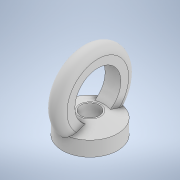
# Autodesk Inventor part: Wire holder
Saved by Autodesk Inventor 2020.2 (Build 242310000, 310)
## iProperties
Created: 2020-01-20
Part Number: Wire holder
Material: Generic
Document SubType Name: Modeling
Designer: Paul Lefeuvre
Density: 1 g/cm^3
Appearance: Default
Author: Paul Lefeuvre
Autodesk Inventor part; units mm, degrees
ref_plane "YZ Plane" through (0, 0, 0) normal (1, 0, 0) x (0, 1, 0)
ref_plane "XZ Plane" through (0, 0, 0) normal (0, 1, 0) x (-1, 0, 0)
ref_plane "XY Plane" through (0, 0, 0) normal (0, 0, 1) x (1, 0, 0)
sketch "Sketch1" plane through (0, 0, 0) normal (1, 0, 0) x (0, 1, 0)
  circle A0 centre (0, 0) radius 12.45
  circle A1 centre (0, 0) radius 20.95
  line L0 (0, 0) -> (-30.2923, 0)
  line L1 (-12.95, 15) -> (-20.95, 15)
  line L2 (-20.95, 15) -> (-20.95, -15)
  line L3 (-20.95, -15) -> (-12.95, -15)
  line L4 (-12.95, 15) -> (-9.5732, 5.7222)
  line L5 (-9.5732, 5.7222) -> (-9.5732, -5.7222)
  line L6 (-9.5732, -5.7222) -> (-12.95, -15)
  line L7 (-9.5732, 5) -> (-20.95, 5)
  line L8 (-20.95, -5) -> (-9.5732, -5)
  point P0 (-9.5732, 0)
  point P1 (-20.95, 0)
  dimension "d0" = 24.9
  dimension "d1" = 8.5
  dimension "d10" = 90
  dimension "d11" = 15
  dimension "d12" = 15
  dimension "d13" = 90
  dimension "d14" = 110
  dimension "d15" = 110
  dimension "d16" = 8
  dimension "d18" = 5
  dimension "d19" = 5
  constraints: 18 end point, 4 point on line, 2 centre point, 2 equal length, 2 perpendicular, 1 coincident, 1 horizontal, 1 tangent, 1 vertical
  measures "d0" diameter of A0
  measures "d1" radial gap between concentric circles of A0 A1
  measures "d10" angle of L1 L2
  measures "d11" distance from line of L1.end L0
  measures "d12" distance from line of L0 L2.end
  measures "d13" angle of L2 L3
  measures "d14" angle of L1 L4
  measures "d15" angle of L3 L6
  measures "d16" distance of L2.end L3.end
  measures "d18" distance between parallel lines of L0 L7
  measures "d19" distance between parallel lines of L0 L8
extrude "Extrusion1" add sketch "Sketch1" along normal mid plane 8.5 contours A0 L4 L1 A1 L3 L6 | A0 L7 A1 L1 L4 | L6 L3 A1 L8 A0 | A0 L0 A1 L7 | L8 A1 L0 A0
fillet "Fillet1" radius 4.25 2 edges at (4.25, -20.95, 0) (-4.25, -20.95, 0)
revolve "Revolution1" add sketch "Sketch1" angle 360 about axis through (0, 0, 0) along (0, -1, 0) contours L6 L3 A1 L8 A0 | A0 L8 L5 L6 | A1 L3 L2 L8
revolve "Revolution2" cut sketch "Sketch1" angle 360 about axis through (0, 0, 0) along (0, -1, 0) contours L8 A1 L0 A0 | A0 L0 L5 L8 | L8 L2 A1
equation "\"d12\" = d11"
equation "\"d15\" = d14"
body "Solid1"
